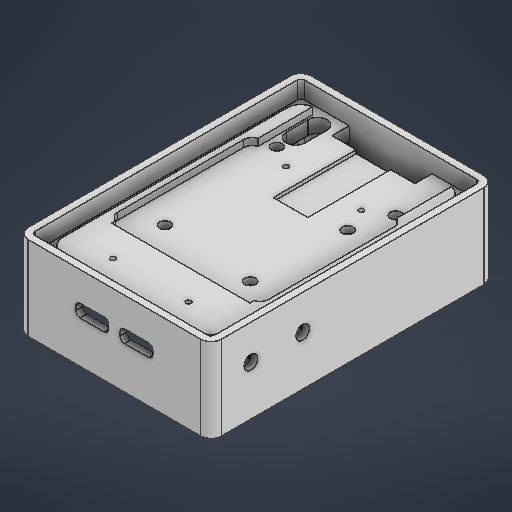
# Autodesk Inventor part: gapura_case_pt1
Saved by Autodesk Inventor 2026.4 (Build 304435000, 435)
## iProperties
Created: 2026-10-02
Part Number: gapura_case_pt1
Material: Generic
Document SubType Name: Modeling
Designer: LENOVO
Density: 1 g/cm^3
Appearance: Default
Author: LENOVO
Autodesk Inventor part; units mm, degrees
ref_plane "YZ Plane" through (0, 0, 0) normal (1, 0, 0) x (0, 1, 0)
ref_plane "XY Plane" through (0, 0, 0) normal (0, 0, 1) x (1, 0, 0)
sketch "Sketch1" plane through (0, 0, 0) normal (0, 1, 0) x (-1, 0, 0)
  line L0 (25, -38) -> (-25, -38)
  line L1 (-25, -38) -> (-25, 38)
  line L2 (-25, 38) -> (25, 38)
  line L3 (25, 38) -> (25, -38)
  line L4 (25, -38) -> (-25, 38) construction
  line L5 (-25, -38) -> (25, 38) construction
  line L6 (-25, -38) -> (-3.5, -38)
  line L7 (-3.5, -38) -> (-3.5, 38)
  line L8 (-3.5, 38) -> (-25, 38)
  line L9 (-25, 38) -> (-25, -38)
  line L10 (-3.5, -38) -> (18, -38)
  line L11 (18, -38) -> (18, 38)
  line L12 (18, 38) -> (-3.5, 38)
  line L13 (-3.5, 38) -> (-3.5, -38)
  line L14 (-25, -39) -> (25, -39)
  line L15 (26, -38) -> (26, 38)
  line L16 (25, 39) -> (-25, 39)
  line L17 (-26, 38) -> (-26, -38)
  line L18 (25, -41) -> (-25, -41)
  line L19 (-28, -38) -> (-28, 38)
  line L20 (-25, 41) -> (25, 41)
  line L21 (28, 38) -> (28, -38)
  arc A0 (25, -39) -> (26, -38) centre (25, -38) ccw
  arc A1 (-26, -38) -> (-25, -39) centre (-25, -38) ccw
  arc A2 (26, 38) -> (25, 39) centre (25, 38) ccw
  arc A3 (-25, 39) -> (-26, 38) centre (-25, 38) ccw
  arc A4 (25, -41) -> (28, -38) centre (25, -38) ccw
  arc A5 (-28, -38) -> (-25, -41) centre (-25, -38) ccw
  arc A6 (-25, 41) -> (-28, 38) centre (-25, 38) ccw
  arc A7 (28, 38) -> (25, 41) centre (25, 38) ccw
  point P0 (0, 0)
  dimension "d0" = 50
  dimension "d1" = 76
  dimension "d2" = 21.5
  dimension "d3" = 21.5
  dimension "d4" = 1
  dimension "d5" = 2
  dimension "d6" = 1
  dimension "d7" = 3
  constraints: 44 end point, 16 point on circle, 16 tangent, 10 parallel, 8 centre point, 6 equal radius, 5 perpendicular, 3 horizontal, 2 midpoint, 2 point on line, 6 other
  measures "d0" distance of L1.end L2.end
  measures "d1" distance of L0.end L1.end
  measures "d2" distance of L8.end L7.end
  measures "d3" distance of L12.end L11.end
  measures "d4" distance between parallel lines of L0 L14
  measures "d5" distance between parallel lines of L14 L18
  measures "d6" radius of A0
  measures "d7" radius of A4
extrude "Extrusion1" add sketch "Sketch1" along normal mid plane 28 contours L18 A5 L19 A6 L20 A7 L21 A4
sketch "Sketch2" plane through (-25, 14, 41) normal (0, 0, 1) x (1, 0, 0)
  line L0 (27.9, -12.4) -> (34.9, -12.4)
  line L1 (35.9, -13.4) -> (35.9, -14.6)
  line L2 (34.9, -15.6) -> (27.9, -15.6)
  line L3 (26.9, -14.6) -> (26.9, -13.4)
  line L4 (26.9, -12.4) -> (35.9, -15.6) construction
  line L5 (35.9, -12.4) -> (26.9, -15.6) construction
  arc A0 (26.9, -14.6) -> (27.9, -15.6) centre (27.9, -14.6) ccw
  arc A1 (27.9, -12.4) -> (26.9, -13.4) centre (27.9, -13.4) ccw
  arc A2 (35.9, -13.4) -> (34.9, -12.4) centre (34.9, -13.4) ccw
  arc A3 (34.9, -15.6) -> (35.9, -14.6) centre (34.9, -14.6) ccw
  line L6 (26.65, -13.4) -> (26.65, -14.6)
  arc A4 (26.65, -14.6) -> (27.9, -15.85) centre (27.9, -14.6) ccw
  line L7 (27.9, -15.85) -> (34.9, -15.85)
  arc A5 (34.9, -15.85) -> (36.15, -14.6) centre (34.9, -14.6) ccw
  line L8 (36.15, -14.6) -> (36.15, -13.4)
  arc A6 (36.15, -13.4) -> (34.9, -12.15) centre (34.9, -13.4) ccw
  line L9 (34.9, -12.15) -> (27.9, -12.15)
  arc A7 (27.9, -12.15) -> (26.65, -13.4) centre (27.9, -13.4) ccw
  line L10 (25, -14) -> (25, -12)
  line L11 (22.1, -12.4) -> (15.1, -12.4)
  line L12 (14.1, -13.4) -> (14.1, -14.6)
  line L13 (15.1, -15.6) -> (22.1, -15.6)
  line L14 (23.1, -14.6) -> (23.1, -13.4)
  line L15 (23.1, -12.4) -> (14.1, -15.6) construction
  line L16 (14.1, -12.4) -> (23.1, -15.6) construction
  arc A8 (22.1, -15.6) -> (23.1, -14.6) centre (22.1, -14.6) ccw
  arc A9 (23.1, -13.4) -> (22.1, -12.4) centre (22.1, -13.4) ccw
  arc A10 (15.1, -12.4) -> (14.1, -13.4) centre (15.1, -13.4) ccw
  arc A11 (14.1, -14.6) -> (15.1, -15.6) centre (15.1, -14.6) ccw
  line L17 (23.35, -13.4) -> (23.35, -14.6)
  arc A12 (22.1, -15.85) -> (23.35, -14.6) centre (22.1, -14.6) ccw
  line L18 (22.1, -15.85) -> (15.1, -15.85)
  arc A13 (13.85, -14.6) -> (15.1, -15.85) centre (15.1, -14.6) ccw
  line L19 (13.85, -14.6) -> (13.85, -13.4)
  arc A14 (15.1, -12.15) -> (13.85, -13.4) centre (15.1, -13.4) ccw
  line L20 (15.1, -12.15) -> (22.1, -12.15)
  arc A15 (23.35, -13.4) -> (22.1, -12.15) centre (22.1, -13.4) ccw
  point P0 (31.4, -14)
  point P1 (18.6, -14)
  dimension "d34" = 9
  dimension "d35" = 3.2
  dimension "d37" = 1
  dimension "d38" = 1.6
  dimension "d39" = 0.25
  dimension "d41" = 2
  dimension "d42" = 1.9
  constraints: 42 end point, 32 point on circle, 25 symmetric about line, 16 centre point, 16 point on line, 8 tangent, 4 parallel, 3 equal radius, 2 midpoint, 2 perpendicular, 2 vertical, 1 coincident, 1 horizontal, 15 other
  measures "d34" distance of L4.end L5.end
  measures "d35" distance of L5.start L4.end
  measures "d37" radius of A0
  measures "d38" distance from line of point (25, -14) L2
  measures "d39" distance between parallel lines of L3 L6
  measures "d41" distance of L10.start L10.end
  measures "d42" distance between parallel lines of L10 L3
extrude "Extrusion2" cut sketch "Sketch2" against normal blind 2 contours L0 A2 L1 A3 L2 A0 L3 A1 | A7 L9 A6 L8 A5 L7 A4 L6 | A9 L14 A8 L13 A11 L12 A10 L11 | L17 A12 L18 A13 L19 A14 L20 A15
sketch "Sketch4" plane through (-25, 14, 41) normal (0, 0, 1) x (1, 0, 0)
  line L0 (34.9, -15.85) -> (27.9, -15.85) projected
  arc A0 (26.65, -14.6) -> (27.9, -15.85) centre (27.9, -14.6) ccw projected
  line L1 (26.65, -14.6) -> (26.65, -13.4) projected
  arc A1 (27.9, -12.15) -> (26.65, -13.4) centre (27.9, -13.4) ccw projected
  line L2 (27.9, -12.15) -> (34.9, -12.15) projected
  arc A2 (36.15, -13.4) -> (34.9, -12.15) centre (34.9, -13.4) ccw projected
  line L3 (36.15, -13.4) -> (36.15, -14.6) projected
  arc A3 (34.9, -15.85) -> (36.15, -14.6) centre (34.9, -14.6) ccw projected
  arc A4 (15.1, -12.15) -> (13.85, -13.4) centre (15.1, -13.4) ccw projected
  line L4 (15.1, -12.15) -> (22.1, -12.15) projected
  arc A5 (23.35, -13.4) -> (22.1, -12.15) centre (22.1, -13.4) ccw projected
  line L5 (23.35, -13.4) -> (23.35, -14.6) projected
  arc A6 (22.1, -15.85) -> (23.35, -14.6) centre (22.1, -14.6) ccw projected
  line L6 (22.1, -15.85) -> (15.1, -15.85) projected
  arc A7 (13.85, -14.6) -> (15.1, -15.85) centre (15.1, -14.6) ccw projected
  line L7 (13.85, -14.6) -> (13.85, -13.4) projected
  line L8 (50, -28) -> (50, 0) projected
  line L9 (0, 0) -> (50, 0) projected
  line L10 (0, 0) -> (0, -28) projected
  line L11 (50, -28) -> (0, -28) projected
  line L12 (11.5, -10.77) -> (38.5, -10.77)
  line L13 (38.5, -10.77) -> (38.5, -12.37)
  line L14 (38.5, -12.37) -> (11.5, -12.37)
  line L15 (11.5, -12.37) -> (11.5, -10.77)
  line L16 (11.5, -10.77) -> (38.5, -12.37) construction
  line L17 (38.5, -10.77) -> (11.5, -12.37) construction
  point P0 (25, -14)
  point P1 (38.4563, -16.1615)
  point P2 (25, -12.42)
  point P3 (25, -11.57)
  dimension "d45" = 0.85
  dimension "d46" = 27
  dimension "d47" = 1.6
  dimension "d48" = 0.05
  dimension "d49" = 1.58
  constraints: 12 end point, 2 midpoint, 2 parallel, 1 horizontal, 1 perpendicular, 1 other
  measures "d45" distance of point (25, -11.57) point (25, -12.42)
  measures "d46" distance of L13.end L14.end
  measures "d47" distance of L12.end L13.end
  measures "d48" distance from line of point (25, -12.42) L14
  measures "d49" distance of point (25, -14) point (25, -12.42)
ref_plane "Work Plane1" through (0, 3.28, 0) normal (0, 1, 0) x (-1, 0, 0)
sketch "Sketch5" plane through (0, 3.28, 0) normal (0, 1, 0) x (-1, 0, 0)
  line L0 (25, 41) -> (-25, 41) projected
  arc A0 (-25, 41) -> (-28, 38) centre (-25, 38) ccw projected
  line L1 (-28, 38) -> (-28, -38) projected
  arc A1 (-28, -38) -> (-25, -41) centre (-25, -38) ccw projected
  line L2 (-25, -41) -> (25, -41) projected
  arc A2 (25, -41) -> (28, -38) centre (25, -38) ccw projected
  line L3 (28, -38) -> (28, 38) projected
  arc A3 (28, 38) -> (25, 41) centre (25, 38) ccw projected
  arc A4 (-26, -38) -> (-25, -39) centre (-25, -38) ccw projected
  line L4 (-26, -38) -> (-26, 38) projected
  arc A5 (-25, 39) -> (-26, 38) centre (-25, 38) ccw projected
  line L5 (-25, 39) -> (25, 39) projected
  arc A6 (26, 38) -> (25, 39) centre (25, 38) ccw projected
  line L6 (26, 38) -> (26, -38) projected
  arc A7 (25, -39) -> (26, -38) centre (25, -38) ccw projected
  line L7 (25, -39) -> (-25, -39) projected
  point P0 (0, 0)
extrude "Extrusion4" add sketch "Sketch5" along normal blind 4 contours L4 A5 L5 A6 L6 A7 L7 A4
sketch "Sketch6" plane through (0, 3.28, 0) normal (0, -1, 0) x (1, 0, 0)
  circle A0 centre (10.9, 30.424) radius 0.75
  line L0 (-25, 39) -> (25, 39) projected
  line L1 (26, 38) -> (26, -38) projected
  circle A1 centre (10.9, -19.576) radius 0.75
  circle A2 centre (-10.9, 30.424) radius 0.75
  circle A3 centre (-10.9, -19.576) radius 0.75
  point P0 (0, 0)
  dimension "d53" = 1.5
  dimension "d54" = 8.576
  dimension "d55" = 10.9
  dimension "d58" = 50
  dimension "d61" = 21.8
  constraints: 4 centre point, 1 horizontal, 1 vertical, 6 other
  measures "d53" diameter of A0
  measures "d54" distance from line of L0 A0.centre
  measures "d55" horizontal distance of point (0, 0) A0.centre
  measures "d58" distance of A0.centre A1.centre
  measures "d61" distance of A0.centre A2.centre
extrude "Extrusion5" cut sketch "Sketch6" against normal blind 4
sketch "Sketch7" plane through (0, 7.28, 0) normal (0, 1, 0) x (1, 0, 0)
  line L0 (-19.555, -21.3) -> (19.555, -21.3)
  line L1 (19.555, -21.3) -> (19.555, 38.7)
  line L2 (19.555, 38.7) -> (-19.555, 38.7)
  line L3 (-19.555, 38.7) -> (-19.555, -21.3)
  line L4 (-8.68, 37.715) -> (-8.68, 35.965)
  line L5 (-8.68, 35.965) -> (-10.43, 35.965)
  line L6 (-10.43, 35.965) -> (-10.43, 37.715)
  line L7 (-10.43, 37.715) -> (-8.68, 37.715)
  circle A0 centre (0.445, 36.84) radius 0.8
  circle A1 centre (7.945, 36.84) radius 0.8
  circle A2 centre (-2.055, 36.84) radius 0.8
  circle A3 centre (-7.055, 36.84) radius 0.8
  circle A4 centre (2.945, 36.84) radius 0.8
  circle A5 centre (5.445, 36.84) radius 0.8
  circle A6 centre (-4.555, 36.84) radius 0.8
  circle A7 centre (12.675, -14.34) radius 1.95
  circle A8 centre (-17.205, 23.25) radius 1.95
  circle A9 centre (17.205, 23.25) radius 1.95
  arc A10 (-19.015, 28.26) -> (-14.595, 28.26) centre (-16.805, 28.26) ccw
  line L8 (-19.015, 28.26) -> (-19.015, 34.59)
  arc A11 (-14.595, 34.59) -> (-19.015, 34.59) centre (-16.805, 34.59) ccw
  line L9 (-14.595, 34.59) -> (-14.595, 28.26)
  arc A12 (-18.565, 28.26) -> (-15.045, 28.26) centre (-16.805, 28.26) ccw
  line L10 (-15.045, 28.26) -> (-15.045, 34.59)
  arc A13 (-15.045, 34.59) -> (-18.565, 34.59) centre (-16.805, 34.59) ccw
  line L11 (-18.565, 34.59) -> (-18.565, 28.26)
  line L12 (-19.555, -21.3) -> (19.555, -21.3)
  line L13 (19.555, -21.3) -> (19.555, 21.3)
  line L14 (19.555, 21.3) -> (-19.555, 21.3)
  line L15 (-19.555, 21.3) -> (-19.555, -21.3)
  arc A14 (-21.35, -18.2) -> (-19.35, -20.2) centre (-19.35, -18.2) ccw
  line L16 (19.35, -20.2) -> (-19.35, -20.2)
  arc A15 (19.35, -20.2) -> (21.35, -18.2) centre (19.35, -18.2) ccw
  line L17 (21.35, 18.2) -> (21.35, -18.2)
  arc A16 (21.35, 18.2) -> (19.35, 20.2) centre (19.35, 18.2) ccw
  line L18 (-19.35, 20.2) -> (19.35, 20.2)
  arc A17 (-19.35, 20.2) -> (-21.35, 18.2) centre (-19.35, 18.2) ccw
  line L19 (-21.35, -18.2) -> (-21.35, 18.2)
  circle A18 centre (-0.53, -11) radius 0.6
  circle A19 centre (-4.23, 14) radius 0.8
  circle A20 centre (5.93, 14) radius 0.8
  circle A21 centre (15.35, -0.88) radius 0.8
  circle A22 centre (0.74, -11) radius 0.6
  circle A23 centre (-5.61, -11) radius 0.6
  circle A24 centre (-13.75, -12.6) radius 2.5
  circle A25 centre (-4.34, -11) radius 0.6
  circle A26 centre (2.01, -11) radius 0.6
  circle A27 centre (15.35, 1.66) radius 0.8
  circle A28 centre (3.39, 14) radius 0.8
  circle A29 centre (-6.77, 14) radius 0.8
  circle A30 centre (-11.85, 14) radius 0.8
  circle A31 centre (-1.69, 14) radius 0.8
  circle A32 centre (13.95, 12.6) radius 2.5
  circle A33 centre (15.35, -3.42) radius 0.8
  circle A34 centre (-1.8, -11) radius 0.6
  circle A35 centre (-6.88, -11) radius 0.6
  circle A36 centre (-8.15, -11) radius 0.6
  circle A37 centre (-3.07, -11) radius 0.6
  circle A38 centre (3.28, -11) radius 0.6
  circle A39 centre (15.35, 4.2) radius 0.8
  circle A40 centre (0.85, 14) radius 0.8
  circle A41 centre (-9.31, 14) radius 0.8
  line L20 (-12, 34) -> (12, 34)
  line L21 (12, 34) -> (12, 39)
  line L22 (12, 39) -> (-12, 39)
  line L23 (-12, 39) -> (-12, 34)
  line L24 (-12, 34) -> (12, 39) construction
  line L25 (12, 34) -> (-12, 39) construction
  line L26 (-25, 39) -> (25, 39) projected
  circle A42 centre (-13.75, -12.6) radius 1.6
  circle A43 centre (-17.205, 23.25) radius 1.6
  circle A44 centre (17.205, 23.25) radius 1.6
  circle A45 centre (13.95, 12.6) radius 1.6
  circle A46 centre (12.675, -14.34) radius 1.6
  arc A47 (-19.515, 28.26) -> (-14.095, 28.26) centre (-16.805, 28.26) ccw
  line L27 (-19.515, 28.26) -> (-19.515, 34.59)
  arc A48 (-14.095, 34.59) -> (-19.515, 34.59) centre (-16.805, 34.59) ccw
  line L28 (-14.095, 34.59) -> (-14.095, 28.26)
  point P0 (0, 0)
  point P1 (0, 8.7)
  point P2 (0, 0)
  point P3 (0, -9.7918)
  point P4 (-21.35, 0)
  point P5 (0, -20.2)
  point P6 (0, 0)
  point P7 (0, 36.5)
  dimension "d66" = 24
  dimension "d67" = 5
  dimension "d69" = 2.5
  dimension "d70" = 3.2
  dimension "d71" = 3.2
  dimension "d72" = 3.2
  dimension "d73" = 3.2
  dimension "d74" = 3.2
  dimension "d75" = 0.5
  constraints: 56 end point, 49 centre point, 20 point on circle, 5 coincident, 4 midpoint, 4 parallel, 2 horizontal, 2 perpendicular, 1 point on line, 3 other
  measures "d66" distance of L22.end L21.end
  measures "d67" distance of L21.end L20.end
  measures "d69" distance from line of point (0, 36.5) L26
  measures "d70" diameter of A42
  measures "d71" diameter of A43
  measures "d72" diameter of A44
  measures "d73" diameter of A45
  measures "d74" diameter of A46
  measures "d75" radial gap between concentric circles of A10 A47
extrude "Extrusion6" cut sketch "Sketch7" against normal blind 4 contours L23 L22 L21 L2 | L2 L21 L20 L23 | L4 L5 L6 L7 | A0 | A1 | A2 | A3 | A4 | A5 | A6 | L8 A11 L9 A10 | L11 A13 L10 A12 | A42 | A43 | A44 | A45 | A46 | L27 A48 L28 A47
sketch "Sketch8" plane through (0, 7.28, 0) normal (0, 1, 0) x (1, 0, 0)
  line L0 (12, 34) -> (-12, 34) projected
  line L1 (5, 10) -> (-5, 10)
  line L2 (-5, 10) -> (-5, 34)
  line L3 (-5, 34) -> (5, 34)
  line L4 (5, 34) -> (5, 10)
  line L5 (5, 10) -> (-5, 34) construction
  line L6 (-5, 10) -> (5, 34) construction
  point P0 (0, 0)
  point P1 (0, 22)
  dimension "d78" = 10
  dimension "d79" = 24
  dimension "d80" = 12.8355
  constraints: 12 end point, 2 midpoint, 2 parallel, 1 horizontal, 1 perpendicular, 1 point on line
  measures "d78" distance of L2.end L3.end
  measures "d79" distance of L3.end L1.start
extrude "Extrusion7" cut sketch "Sketch8" against normal blind 3
sketch "Sketch9" plane through (0, 7.28, 0) normal (0, 1, 0) x (1, 0, 0)
  line L0 (-25, -41) -> (25, -41) projected
  arc A0 (25, -41) -> (28, -38) centre (25, -38) ccw projected
  line L1 (28, -38) -> (28, 38) projected
  arc A1 (28, 38) -> (25, 41) centre (25, 38) ccw projected
  line L2 (25, 41) -> (-25, 41) projected
  arc A2 (-25, 41) -> (-28, 38) centre (-25, 38) ccw projected
  line L3 (-28, 38) -> (-28, -38) projected
  arc A3 (-28, -38) -> (-25, -41) centre (-25, -38) ccw projected
  arc A4 (26, 38) -> (25, 39) centre (25, 38) ccw projected
  line L4 (26, 38) -> (26, -38) projected
  arc A5 (25, -39) -> (26, -38) centre (25, -38) ccw projected
  line L5 (25, -39) -> (-25, -39) projected
  arc A6 (-26, -38) -> (-25, -39) centre (-25, -38) ccw projected
  line L6 (-26, -38) -> (-26, 38) projected
  arc A7 (-25, 39) -> (-26, 38) centre (-25, 38) ccw projected
  line L7 (-25, 39) -> (25, 39) projected
  line L8 (26, 39) -> (-26, 39)
  line L9 (-26, 39) -> (-26, -39)
  line L10 (-26, -39) -> (26, -39)
  line L11 (26, -39) -> (26, 39)
  line L12 (26, 39) -> (-26, -39) construction
  line L13 (-26, 39) -> (26, -39) construction
  line L14 (19.5, -36.5) -> (-19.5, -36.5)
  line L15 (-23.5, -32.5) -> (-23.5, 32.5)
  line L16 (-19.5, 36.5) -> (19.5, 36.5)
  line L17 (23.5, 32.5) -> (23.5, -32.5)
  arc A8 (-23.5, -32.5) -> (-19.5, -36.5) centre (-19.5, -32.5) ccw
  arc A9 (-19.5, 36.5) -> (-23.5, 32.5) centre (-19.5, 32.5) ccw
  arc A10 (23.5, 32.5) -> (19.5, 36.5) centre (19.5, 32.5) ccw
  arc A11 (19.5, -36.5) -> (23.5, -32.5) centre (19.5, -32.5) ccw
  point P0 (0, 0)
  dimension "d83" = 52
  dimension "d84" = 78
  dimension "d85" = 2.5
  dimension "d86" = 4
  constraints: 20 end point, 8 point on circle, 8 tangent, 4 centre point, 4 parallel, 3 equal radius, 2 midpoint, 2 perpendicular, 1 horizontal, 3 other
  measures "d83" distance of L10.end L9.end
  measures "d84" distance of L9.end L8.end
  measures "d85" distance between parallel lines of L10 L14
  measures "d86" radius of A8
extrude "Extrusion8" cut sketch "Sketch9" against normal blind 2 contours L4 A5 L5 A6 L6 A7 L7 A4
sketch "Sketch10" plane through (25, -14, 39) normal (0, 0, -1) x (-1, 0, 0)
  line L0 (34.9, 12.15) -> (27.9, 12.15)
  arc A0 (26.65, 13.4) -> (27.9, 12.15) centre (27.9, 13.4) ccw
  line L1 (26.65, 13.4) -> (26.65, 14.6)
  arc A1 (27.9, 15.85) -> (26.65, 14.6) centre (27.9, 14.6) ccw
  line L2 (27.9, 15.85) -> (34.9, 15.85)
  arc A2 (36.15, 14.6) -> (34.9, 15.85) centre (34.9, 14.6) ccw
  line L3 (36.15, 14.6) -> (36.15, 13.4)
  arc A3 (34.9, 12.15) -> (36.15, 13.4) centre (34.9, 13.4) ccw
  arc A4 (15.1, 15.85) -> (13.85, 14.6) centre (15.1, 14.6) ccw
  line L4 (15.1, 15.85) -> (22.1, 15.85)
  arc A5 (23.35, 14.6) -> (22.1, 15.85) centre (22.1, 14.6) ccw
  line L5 (23.35, 14.6) -> (23.35, 13.4)
  arc A6 (22.1, 12.15) -> (23.35, 13.4) centre (22.1, 13.4) ccw
  line L6 (22.1, 12.15) -> (15.1, 12.15)
  arc A7 (13.85, 13.4) -> (15.1, 12.15) centre (15.1, 13.4) ccw
  line L7 (13.85, 13.4) -> (13.85, 14.6)
  line L8 (53.2452, 6.0903) -> (53.2452, 34.0903)
  line L9 (3.2452, 34.0903) -> (53.2452, 34.0903)
  line L10 (3.2452, 34.0903) -> (3.2452, 6.0903)
  line L11 (53.2452, 6.0903) -> (3.2452, 6.0903)
  line L12 (11.5, 17.23) -> (38.5, 17.23)
  line L13 (38.5, 17.23) -> (38.5, 15.63)
  line L14 (38.5, 15.63) -> (11.5, 15.63)
  line L15 (11.5, 15.63) -> (11.5, 17.23)
  line L16 (11.5, 17.23) -> (38.5, 15.63) construction
  line L17 (38.5, 17.23) -> (11.5, 15.63) construction
  line L18 (50, 17.28) -> (0, 17.28) projected
  line L19 (11.5, 17.23) -> (38.5, 17.23)
  line L20 (38.5, 17.23) -> (38.5, 17.28)
  line L21 (38.5, 17.28) -> (11.5, 17.28)
  line L22 (11.5, 17.28) -> (11.5, 17.23)
  point P0 (25, 14)
  point P1 (25, 14)
  point P2 (38.4563, 11.8385)
  point P3 (25, 15.58)
  point P4 (25, 16.43)
  dimension "d89" = 0.85
  dimension "d90" = 27
  dimension "d91" = 1.6
  dimension "d92" = 0.05
  dimension "d93" = 1.58
  constraints: 44 end point, 16 point on circle, 8 centre point, 4 parallel, 2 horizontal, 2 midpoint, 2 perpendicular, 1 point on line
  measures "d89" distance of point (25, 16.43) point (25, 15.58)
  measures "d90" distance of L13.end L14.end
  measures "d91" distance of L12.end L13.end
  measures "d92" distance from line of point (25, 15.58) L14
  measures "d93" distance of point (25, 14) point (25, 15.58)
extrude "Extrusion10" cut sketch "Sketch10" against normal blind 1.5 contours L14 A1 L2 A2 | A2 L2 A1 L14 A5 L4 A4 L15 L12 L13 | L14 A4 L4 A5 | L12 L22 L18 L20
sketch "Sketch11" plane through (0, 3.28, 0) normal (0, -1, 0) x (1, 0, 0)
  line L0 (-12.7055, 39) -> (12.7055, 39)
  line L1 (12.7055, 39) -> (12.7055, -21.376)
  line L2 (12.7055, -21.376) -> (-12.7055, -21.376)
  line L3 (-12.7055, -21.376) -> (-12.7055, 39)
  line L4 (-12.7055, 39) -> (12.7055, -21.376) construction
  line L5 (12.7055, 39) -> (-12.7055, -21.376) construction
  line L6 (-25, 39) -> (25, 39) projected
  line L7 (-12, -39) -> (-12, -34) projected
  line L8 (-12, -34) -> (12, -34) projected
  line L9 (12, -34) -> (12, -39) projected
  line L10 (25, -39) -> (12, -39) projected
  arc A0 (25, -39) -> (26, -38) centre (25, -38) ccw projected
  line L11 (26, 38) -> (26, -38) projected
  arc A1 (26, 38) -> (25, 39) centre (25, 38) ccw projected
  line L12 (13.5, 39) -> (25, 39) projected
  line L13 (13.5, 39) -> (13.5, 40.5) projected
  line L14 (13.5, 40.5) -> (-13.5, 40.5) projected
  line L15 (-13.5, 39) -> (-13.5, 40.5) projected
  line L16 (-25, 39) -> (-13.5, 39) projected
  arc A2 (-25, 39) -> (-26, 38) centre (-25, 38) ccw projected
  line L17 (-26, -38) -> (-26, 38) projected
  arc A3 (-26, -38) -> (-25, -39) centre (-25, -38) ccw projected
  line L18 (-12, -39) -> (-25, -39) projected
  circle A4 centre (10.9, 30.424) radius 0.75 projected
  circle A5 centre (-10.9, -19.576) radius 0.75 projected
  circle A6 centre (-10.9, 30.424) radius 0.75 projected
  circle A7 centre (10.9, -19.576) radius 0.75 projected
  circle A8 centre (-13.75, 12.6) radius 1.6 projected
  circle A9 centre (-17.205, -23.25) radius 1.6 projected
  arc A10 (-14.095, -28.26) -> (-19.515, -28.26) centre (-16.805, -28.26) ccw projected
  line L19 (-14.095, -28.26) -> (-14.095, -34.59) projected
  arc A11 (-19.515, -34.59) -> (-14.095, -34.59) centre (-16.805, -34.59) ccw projected
  line L20 (-19.515, -34.59) -> (-19.515, -28.26) projected
  circle A12 centre (12.675, 14.34) radius 1.6 projected
  circle A13 centre (17.205, -23.25) radius 1.6 projected
  circle A14 centre (13.95, -12.6) radius 1.6 projected
  line L21 (-13.2055, 39.5) -> (13.2055, 39.5)
  line L22 (13.2055, 39.5) -> (13.2055, -21.876)
  line L23 (13.2055, -21.876) -> (-13.2055, -21.876)
  line L24 (-13.2055, -21.876) -> (-13.2055, 39.5)
  line L25 (26, 33) -> (21.8, 33)
  line L26 (21.8, 33) -> (21.8, 26)
  line L27 (21.8, 26) -> (26, 26)
  line L28 (26, 26) -> (26, 33)
  line L29 (26, 18) -> (21.73, 18)
  line L30 (21.73, 18) -> (21.73, 11)
  line L31 (21.73, 11) -> (26, 11)
  line L32 (26, 11) -> (26, 18)
  line L33 (-13.5, 39) -> (-13.5, 40.5) projected
  line L34 (-13.5, 39) -> (13.5, 39)
  line L35 (13.5, 39) -> (13.5, -21.876)
  line L36 (13.5, -21.876) -> (-13.5, -21.876)
  line L37 (-13.5, -21.876) -> (-13.5, 39)
  point P0 (0, 0)
  point P1 (0, 8.812)
  point P2 (25, 39)
  point P3 (13.5, 15.7109)
  point P4 (13.5, 12.9691)
  point P5 (13.5, -11.0646)
  point P6 (13.5, -14.1354)
  point P7 (13.2055, -21.876)
  point P8 (-13.2055, -21.876)
  point P9 (-13.5, 11.0197)
  point P10 (-13.5, 14.1803)
  dimension "d98" = 25.411
  dimension "d99" = 60.376
  dimension "d100" = 30.188
  dimension "d101" = 0.5
  dimension "d108" = 4.2
  dimension "d109" = 7
  dimension "d110" = 4.27
  dimension "d111" = 7
  dimension "d112" = 8
  dimension "d113" = 6
  dimension "d114" = 27
  constraints: 44 end point, 10 parallel, 5 perpendicular, 4 horizontal, 2 midpoint, 2 point on line, 3 other
  measures "d98" distance of L1.end L2.end
  measures "d99" distance of L0.end L1.end
  measures "d100" distance from line of L6 point (0, 8.812)
  measures "d101" distance between parallel lines of L3 L24
  measures "d108" distance of L27.end L26.end
  measures "d109" distance of L26.end L25.end
  measures "d110" distance of L31.end L30.end
  measures "d111" distance of L29.end L30.end
  measures "d112" distance between parallel lines of L27 L29
  measures "d113" distance between parallel lines of L6 L25
  measures "d114" distance of L35.end L36.end
extrude "Extrusion11" add sketch "Sketch11" along normal blind 2 contours L37 A8 L36 L23 L35 A14 A12 L6 A1 L11 L25 L26 L27 L29 L30 L31 A0 L10 L9 L8 L7 L18 A3 L17 A2
sketch "Sketch13" plane through (26, -14, -38) normal (-1, 0, 0) x (0, 0, 1)
  line L0 (49, 15.28) -> (0, 15.28) projected
  line L1 (0, 0) -> (0, 15.28) projected
  line L2 (76, 0) -> (0, 0) projected
  line L3 (76, 0) -> (76, 15.28) projected
  line L4 (76, 15.28) -> (71, 15.28) projected
  line L5 (71, 15.28) -> (71, 17.28) projected
  line L6 (71, 17.28) -> (64, 17.28) projected
  line L7 (64, 17.28) -> (64, 15.28) projected
  line L8 (64, 15.28) -> (56, 15.28) projected
  line L9 (56, 15.28) -> (56, 17.28) projected
  line L10 (56, 17.28) -> (49, 17.28) projected
  line L11 (49, 17.28) -> (49, 15.28) projected
  circle A0 centre (67.5, 14.28) radius 2
  circle A1 centre (52.5, 14.28) radius 2
  point P0 (38, 14)
  point P1 (67.5, 17.28)
  point P2 (52.5, 17.28)
  dimension "d117" = 3
  dimension "d118" = 4
  constraints: 2 centre point, 2 coincident, 2 midpoint
  measures "d117" distance from line of L6 point (67.5, 14.28)
  measures "d118" diameter of A0
extrude "Extrusion12" cut sketch "Sketch13" against normal blind 2 contours A0 | A1
sketch "Sketch14" plane through (0, 1.28, 0) normal (0, -1, 0) x (1, 0, 0)
  line L0 (26, 11) -> (26, -38) projected
  line L1 (26, 11) -> (21.73, 11) projected
  line L2 (21.73, 11) -> (21.73, 18) projected
  line L3 (21.73, 18) -> (26, 18) projected
  line L4 (26, 26) -> (26, 18) projected
  line L5 (26, 26) -> (21.8, 26) projected
  line L6 (21.8, 26) -> (21.8, 33) projected
  line L7 (21.8, 33) -> (26, 33) projected
  line L8 (26, 38) -> (26, 33) projected
  arc A0 (26, 38) -> (25, 39) centre (25, 38) ccw projected
  line L9 (13.5, 39) -> (25, 39) projected
  line L10 (13.5, 39) -> (13.5, 15.7109) projected
  arc A1 (13.5, 12.9691) -> (13.5, 15.7109) centre (12.675, 14.34) ccw projected
  line L11 (13.5, 12.9691) -> (13.5, -11.0646) projected
  arc A2 (13.5, -14.1354) -> (13.5, -11.0646) centre (13.95, -12.6) ccw projected
  line L12 (13.5, -14.1354) -> (13.5, -21.876) projected
  line L13 (13.5, -21.876) -> (-13.5, -21.876) projected
  line L14 (-13.5, -21.876) -> (-13.5, 11.0197) projected
  arc A3 (-13.5, 14.1803) -> (-13.5, 11.0197) centre (-13.75, 12.6) ccw projected
  line L15 (-13.5, 14.1803) -> (-13.5, 39) projected
  line L16 (-25, 39) -> (-13.5, 39) projected
  arc A4 (-25, 39) -> (-26, 38) centre (-25, 38) ccw projected
  line L17 (-26, -38) -> (-26, 38) projected
  arc A5 (-26, -38) -> (-25, -39) centre (-25, -38) ccw projected
  line L18 (-12, -39) -> (-25, -39) projected
  line L19 (-12, -39) -> (-12, -34) projected
  line L20 (-12, -34) -> (12, -34) projected
  line L21 (12, -34) -> (12, -39) projected
  line L22 (25, -39) -> (12, -39) projected
  arc A6 (25, -39) -> (26, -38) centre (25, -38) ccw projected
  circle A7 centre (-17.205, -23.25) radius 1.6 projected
  circle A8 centre (17.205, -23.25) radius 1.6 projected
  line L23 (-19.515, -34.59) -> (-19.515, -28.26) projected
  arc A9 (-14.095, -28.26) -> (-19.515, -28.26) centre (-16.805, -28.26) ccw projected
  line L24 (-14.095, -28.26) -> (-14.095, -34.59) projected
  arc A10 (-19.515, -34.59) -> (-14.095, -34.59) centre (-16.805, -34.59) ccw projected
  line L25 (26, 26) -> (21.73, 26)
  line L26 (21.73, 26) -> (21.73, 18)
  line L27 (21.73, 18) -> (26, 18)
  line L28 (26, 18) -> (26, 26)
  line L29 (21.8, 33) -> (26, 33)
  line L30 (26, 33) -> (26, 39)
  line L31 (26, 39) -> (21.8, 39)
  line L32 (21.8, 39) -> (21.8, 33)
  line L33 (21.73, 11) -> (26, 11)
  line L34 (26, 11) -> (26, 8.5)
  line L35 (26, 8.5) -> (21.73, 8.5)
  line L36 (21.73, 8.5) -> (21.73, 11)
  point P0 (0, 0)
  dimension "d121" = 2.5
  constraints: 24 end point, 6 parallel, 3 horizontal, 3 perpendicular, 2 point on line
  measures "d121" distance of L33.end L34.end
extrude "Extrusion13" add sketch "Sketch14" along normal blind 4 contours L0 L35 L36 L1 | L26 L25 L5 L4 L3 | L32 L9 A0 L8 L7
sketch "Sketch15" plane through (0, 7.28, 0) normal (0, 1, 0) x (1, 0, 0)
  line L0 (-19.555, -21.3) -> (19.555, -21.3)
  line L1 (19.555, -21.3) -> (19.555, 38.7)
  line L2 (19.555, 38.7) -> (-19.555, 38.7)
  line L3 (-19.555, 38.7) -> (-19.555, -21.3)
  line L4 (-19.555, -21.3) -> (19.555, -21.3)
  line L5 (19.555, -21.3) -> (19.555, 21.3)
  line L6 (19.555, 21.3) -> (-19.555, 21.3)
  line L7 (-19.555, 21.3) -> (-19.555, -21.3)
  arc A0 (-21.35, -18.2) -> (-19.35, -20.2) centre (-19.35, -18.2) ccw
  line L8 (19.35, -20.2) -> (-19.35, -20.2)
  arc A1 (19.35, -20.2) -> (21.35, -18.2) centre (19.35, -18.2) ccw
  line L9 (21.35, 18.2) -> (21.35, -18.2)
  arc A2 (21.35, 18.2) -> (19.35, 20.2) centre (19.35, 18.2) ccw
  line L10 (-19.35, 20.2) -> (19.35, 20.2)
  arc A3 (-19.35, 20.2) -> (-21.35, 18.2) centre (-19.35, 18.2) ccw
  line L11 (-21.35, -18.2) -> (-21.35, 18.2)
  line L12 (-12, 34) -> (12, 34)
  line L13 (12, 34) -> (12, 39)
  line L14 (12, 39) -> (-12, 39)
  line L15 (-12, 39) -> (-12, 34)
  line L16 (-12, 34) -> (12, 39) construction
  line L17 (12, 34) -> (-12, 39) construction
  line L18 (-25, 39) -> (25, 39)
  arc A4 (21.85, 18.2) -> (19.35, 20.7) centre (19.35, 18.2) ccw
  line L19 (21.85, 18.2) -> (21.85, -18.2)
  arc A5 (19.35, -20.7) -> (21.85, -18.2) centre (19.35, -18.2) ccw
  line L20 (19.35, -20.7) -> (-19.35, -20.7)
  arc A6 (-21.85, -18.2) -> (-19.35, -20.7) centre (-19.35, -18.2) ccw
  line L21 (-21.85, -18.2) -> (-21.85, 18.2)
  arc A7 (-19.35, 20.7) -> (-21.85, 18.2) centre (-19.35, 18.2) ccw
  line L22 (-19.35, 20.7) -> (19.35, 20.7)
  line L23 (20.055, 39.2) -> (20.055, -21.8)
  line L24 (20.055, -21.8) -> (-20.055, -21.8)
  line L25 (-20.055, -21.8) -> (-20.055, 39.2)
  line L26 (-20.055, 39.2) -> (20.055, 39.2)
  line L27 (25, -41) -> (-25, -41) projected
  arc A8 (-28, -38) -> (-25, -41) centre (-25, -38) ccw projected
  line L28 (-28, -38) -> (-28, 38) projected
  arc A9 (-25, 41) -> (-28, 38) centre (-25, 38) ccw projected
  line L29 (-25, 41) -> (25, 41) projected
  arc A10 (28, 38) -> (25, 41) centre (25, 38) ccw projected
  line L30 (28, 38) -> (28, -38) projected
  arc A11 (25, -41) -> (28, -38) centre (25, -38) ccw projected
  arc A12 (26, 38) -> (25, 39) centre (25, 38) ccw projected
  line L31 (25, 39) -> (-25, 39) projected
  arc A13 (-25, 39) -> (-26, 38) centre (-25, 38) ccw projected
  line L32 (-26, 38) -> (-26, -38) projected
  arc A14 (-26, -38) -> (-25, -39) centre (-25, -38) ccw projected
  line L33 (-25, -39) -> (25, -39) projected
  arc A15 (25, -39) -> (26, -38) centre (25, -38) ccw projected
  line L34 (26, -38) -> (26, 38) projected
  point P0 (0, 0)
  point P1 (0, 0)
  point P2 (0, 8.7)
  point P3 (0, 0)
  point P4 (-21.35, 0)
  point P5 (0, -20.2)
  point P6 (0, 0)
  point P7 (20.055, 20.5985)
  point P8 (-20.055, 20.5985)
  point P9 (-20.055, -20.5985)
  point P10 (20.055, -20.5985)
  point P11 (20.055, 39)
  point P12 (-20.055, 39)
  dimension "d124" = 24
  dimension "d125" = 5
  dimension "d133" = 0.5
  dimension "d134" = 0.5
  constraints: 54 end point, 16 point on circle, 8 centre point, 4 parallel, 2 horizontal, 2 midpoint, 2 perpendicular, 1 point on line, 10 other
  measures "d124" distance of L14.end L13.end
  measures "d125" distance of L13.end L12.end
  measures "d133" radial gap between concentric circles of A2 A4
  measures "d134" distance between parallel lines of L1 L23
extrude "Extrusion14" cut sketch "Sketch15" against normal blind 2 contours L3 A6 L20 A5 L1 L0 | L0 L1 A5 L23 L24 L25 A6 L3 | A6 L25 A0 L3 | L3 A0 L8 A1 L1 A5 L20 A6 | L1 A1 L23 A5 | A0 L25 A3 L3 | L3 A3 L10 A2 L1 A1 L8 A0 | A6 L21 A7 L25 A3 L11 A0 | L1 A2 L23 A1 | L23 A1 L9 A2 A4 L19 A5 | A3 L25 A7 L3 | L3 A7 L22 A4 L1 A2 L10 A3 | A0 L11 A3 L25 | L1 A4 L23 A2 | L23 A2 L9 A1 | A7 L25 L18 L15 L2 L3 | L3 L6 L1 A4 L22 A7 | L1 L2 L13 L18 L23 A4 | L3 L2 L15 L12 L13 L1 L6
sketch "Sketch16" plane through (0, 14, 0) normal (0, 1, 0) x (1, 0, 0)
  line L0 (-25, -41) -> (25, -41) projected
  arc A0 (25, -41) -> (28, -38) centre (25, -38) ccw projected
  line L1 (28, -38) -> (28, 38) projected
  arc A1 (28, 38) -> (25, 41) centre (25, 38) ccw projected
  line L2 (25, 41) -> (-25, 41) projected
  arc A2 (-25, 41) -> (-28, 38) centre (-25, 38) ccw projected
  line L3 (-28, 38) -> (-28, -38) projected
  arc A3 (-28, -38) -> (-25, -41) centre (-25, -38) ccw projected
  arc A4 (26, 38) -> (25, 39) centre (25, 38) ccw projected
  line L4 (26, 38) -> (26, -38) projected
  arc A5 (25, -39) -> (26, -38) centre (25, -38) ccw projected
  line L5 (25, -39) -> (-25, -39) projected
  arc A6 (-26, -38) -> (-25, -39) centre (-25, -38) ccw projected
  line L6 (-26, -38) -> (-26, 38) projected
  arc A7 (-25, 39) -> (-26, 38) centre (-25, 38) ccw projected
  line L7 (-25, 39) -> (25, 39) projected
  point P0 (0, 0)
extrude "Extrusion15" cut sketch "Sketch16" against normal blind 3.72
equation "\"d38\" = 0.5 * d35"
equation "\"d61\" = 2 * d55"
equation "\"d69\" = 0.5 * d67"
equation "\"d100\" = 0.5 * d99"
body "Solid1"
